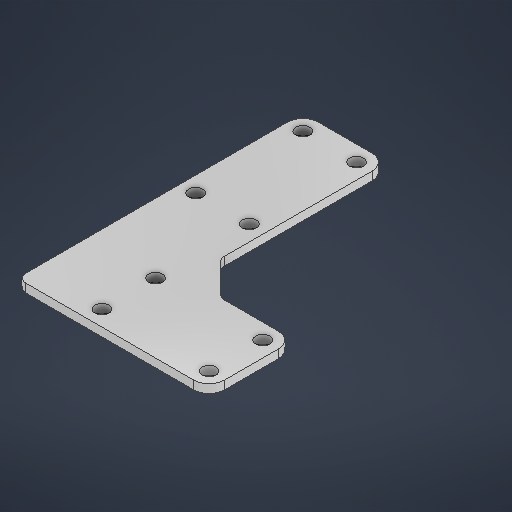
# Autodesk Inventor part: CNC-013-ZAxisMainMount
Saved by Autodesk Inventor 2026.2 (Build 302298000, 298)
## iProperties
Created: 2026-06-19
Part Number: CNC-013-ZAxisMainMount
Material: Aluminum 6061
Document SubType Name: Modeling
Designer: Kenji
Density: 2.7 g/cm^3
Appearance: Aluminum - Dark
Author: Kenji
Autodesk Inventor part; units mm, degrees
ref_plane "YZ Plane" through (0, 0, 0) normal (1, 0, 0) x (0, 1, 0)
ref_plane "XZ Plane" through (0, 0, 0) normal (0, 1, 0) x (-1, 0, 0)
ref_plane "XY Plane" through (0, 0, 0) normal (0, 0, 1) x (1, 0, 0)
sketch "Sketch1" plane through (0, 0, 0) normal (0, 1, 0) x (-1, 0, 0)
  circle A0 centre (0, 0) radius 2.63
  line L0 (0, 0) -> (0, -2.63) construction
  line L1 (0, 0) -> (-2.63, 0) construction
  circle A1 centre (0, -20) radius 2.63
  circle A2 centre (-20, 0) radius 2.63 construction
  circle A3 centre (-20, -20) radius 2.63 construction
  circle A4 centre (-40, 0) radius 2.63
  circle A5 centre (-40, -20) radius 2.63
  circle A6 centre (0, -55) radius 2.63
  circle A7 centre (20, -55) radius 2.63
  circle A8 centre (20, -95) radius 2.63
  circle A9 centre (0, -95) radius 2.63
  circle A10 centre (0, 0) radius 5.805 construction
  circle A11 centre (20, -55) radius 5.805 construction
  circle A12 centre (0, -55) radius 5.805 construction
  circle A13 centre (20, -95) radius 5.805 construction
  circle A14 centre (0, -95) radius 5.805 construction
  circle A15 centre (-40, -20) radius 5.805 construction
  circle A16 centre (-40, 0) radius 5.805 construction
  line L2 (25.805, -95) -> (25.805, 2.63)
  line L3 (22.63, 5.805) -> (-40, 5.805)
  line L4 (-45.805, 0) -> (-45.805, -20)
  line L5 (-19.8201, -25.805) -> (-40, -25.805)
  circle A17 centre (-20, -20) radius 5.805 construction
  line L6 (-5.805, -39.8201) -> (-5.805, -95)
  line L7 (20, -100.805) -> (0, -100.805)
  arc A18 (20, -100.805) -> (25.805, -95) centre (20, -95) ccw
  arc A19 (-5.805, -95) -> (0, -100.805) centre (0, -95) ccw
  arc A20 (-45.805, -20) -> (-40, -25.805) centre (-40, -20) ccw
  arc A21 (-40, 5.805) -> (-45.805, 0) centre (-40, 0) ccw
  line L8 (-6.7349, -37.5751) -> (-17.5751, -26.7349)
  arc A22 (-5.805, -39.8201) -> (-6.7349, -37.5751) centre (-8.98, -39.8201) ccw
  arc A23 (-17.5751, -26.7349) -> (-19.8201, -25.805) centre (-19.8201, -28.98) ccw
  arc A24 (25.805, 2.63) -> (22.63, 5.805) centre (22.63, 2.63) ccw
  point P0 (0, -22.63)
  point P1 (-2.63, -20)
  point P2 (-20, -2.63)
  point P3 (-22.63, 0)
  point P4 (-20, -22.63)
  point P5 (-22.63, -20)
  point P6 (-40, -2.63)
  point P7 (-42.63, 0)
  point P8 (-40, -22.63)
  point P9 (-42.63, -20)
  point P10 (-5.805, -25.805)
  point P11 (-5.805, -38.505)
  point P12 (-18.505, -25.805)
  dimension "d0" = 5.26
  dimension "d3" = 20
  dimension "d6" = 20
  dimension "d10" = 20
  dimension "d12" = 75
  dimension "d13" = 40
  dimension "d14" = 3.175
  dimension "d16" = 12.7
  dimension "d17" = 12.7
  dimension "d18" = 3.175
  constraints: 34 point on circle, 25 centre point, 20 tangent, 18 end point, 16 equal radius, 8 coincident, 6 point on line, 3 vertical, 3 vertical alignment, 2 horizontal alignment, 1 horizontal, 1 perpendicular, 20 other
  measures "d0" diameter of A0
  measures "d3" distance of L0.start A1.centre
  measures "d6" distance of L0.start A2.centre
  measures "d10" distance of A7.centre A6.centre
  measures "d12" distance of A9.centre A1.centre
  measures "d13" distance of A9.centre A6.centre
  measures "d14" radial gap between concentric circles of A10 A0
  measures "d16" distance of point (-5.805, -38.505) point (-5.805, -25.805)
  measures "d17" distance of point (-18.505, -25.805) point (-5.805, -25.805)
  measures "d18" radius of A22
extrude "Extrusion1" add sketch "Sketch1" along normal blind 3.175
equation "\"d17\" = d16"
body "Solid1"
